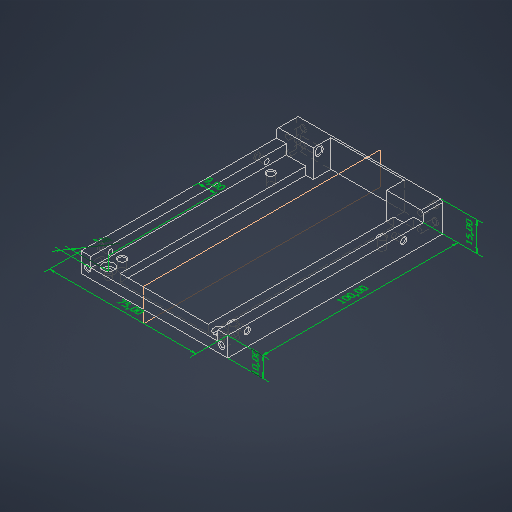
# Autodesk Inventor part: podstawa
Saved by Autodesk Inventor 2026.1 (Build 301233020, 233B)
## iProperties
Created: 2025-11-03
Part Number: podstawa
Material: Stainless Steel, Polished
Document SubType Name: Modeling
Designer: Jan
Density: 8 g/cm^3
Appearance: Stainless - Polished
Author: Jan
Autodesk Inventor part; units mm, degrees
ref_plane "YZ Plane" through (0, 0, 0) normal (1, 0, 0) x (0, 1, 0)
ref_plane "XZ Plane" through (0, 0, 0) normal (0, 1, 0) x (-1, 0, 0)
ref_plane "XY Plane" through (0, 0, 0) normal (0, 0, 1) x (1, 0, 0)
sketch "Sketch1" plane through (0, 0, 0) normal (0, 1, 0) x (-1, 0, 0)
  line L0 (37.5, 55) -> (-37.5, 55)
  line L1 (-37.5, 55) -> (-37.5, -55)
  line L2 (-37.5, -55) -> (37.5, -55)
  line L3 (37.5, -55) -> (37.5, 55)
  point P0 (0, 0)
  point P1 (0, 55)
  dimension "d1" = 75
  dimension "d2" = 37.5
  dimension "d3" = 55
  dimension "d125" = 55
  dimension "d126" = 110
  constraints: 8 end point, 2 parallel, 1 horizontal, 1 midpoint, 1 perpendicular
  measures "d1" distance of L1.end L2.end
  measures "d2" distance from line of point (0, 0) L1
  measures "d3" distance of point (0, 55) point (0, 0)
  measures "d125" distance from line of point (0, 0) L0
  measures "d126" distance of L2.end L0.start
extrude "Extrusion1" add sketch "Sketch1" along normal blind 5
sketch "Sketch2" plane through (0, 5, 0) normal (0, 1, 0) x (1, 0, 0)
  line L0 (37.5, -55) -> (37.5, 55) projected
  line L1 (37.5, -55) -> (37.5, 55)
  line L2 (37.5, 55) -> (-37.5, 55)
  line L3 (-37.5, 55) -> (-37.5, -55) projected
  line L4 (-37.5, 55) -> (-37.5, -55)
  line L5 (-37.5, -55) -> (37.5, -55) projected
  line L6 (-37.5, -55) -> (-32.5, -55)
  line L7 (-32.5, -55) -> (-32.5, 45)
  line L8 (-32.5, 45) -> (-37.5, 45)
  line L9 (-37.5, 45) -> (-37.5, -55)
  line L10 (37.5, -55) -> (32.5, -55)
  line L11 (32.5, -55) -> (32.5, 45)
  line L12 (32.5, 45) -> (37.5, 45)
  line L13 (37.5, 45) -> (37.5, -55)
  point P0 (37.5, 45)
  point P1 (-37.5, 45)
  dimension "d13" = 5
  dimension "d14" = 100
  dimension "d15" = 5
  constraints: 22 end point, 6 equal length, 3 perpendicular, 2 horizontal
  measures "d13" distance of L8.end L7.end
  measures "d14" distance of L6.end L7.end
  measures "d15" distance of L11.end L12.end
extrude "Extrusion2" add sketch "Sketch2" along normal blind 5 contours L5 L11 L12 L0 | L5 L3 L8 L7
sketch "Sketch3" plane through (0, 5, 0) normal (0, 1, 0) x (1, 0, 0)
  line L0 (-37.5, 55) -> (37.5, 55)
  line L1 (37.5, 55) -> (37.5, 45)
  line L2 (37.5, 45) -> (-37.5, 45)
  line L3 (-37.5, 45) -> (-37.5, 55)
  point P0 (0, 0)
  constraints: 8 end point, 2 parallel, 1 horizontal, 1 perpendicular
extrude "Extrusion3" add sketch "Sketch3" along normal blind 10
chamfer "Chamfer2" distance 1 angle 45 1 edges at (-37.5, 15, -50)
chamfer "Chamfer3" distance 1 angle 45 1 edges at (37.5, 15, -50)
sketch "Sketch5" plane through (-32.5, 5, -45) normal (0, 0, 1) x (1, 0, 0)
  line L0 (-4, 10) -> (69, 10) projected
  line L1 (13.75, 10) -> (51.25, 10)
  line L2 (51.25, 10) -> (51.25, 0)
  line L3 (51.25, 0) -> (13.75, 0)
  line L4 (13.75, 0) -> (13.75, 10)
  line L5 (65, 0) -> (0, 0) projected
  line L6 (-5, 5) -> (-5, 9) projected
  point P0 (32.5, -5)
  point P1 (70, 5)
  point P2 (70, 9)
  dimension "d46" = 37.5
  dimension "d47" = 10
  dimension "d48" = 10
  dimension "d49" = 18.75
  dimension "d50" = 75
  dimension "d51" = 18.75
  constraints: 8 end point, 2 parallel, 1 horizontal, 1 perpendicular, 1 point on line
  measures "d46" distance of L2.end L3.end
  measures "d47" distance of L1.start L3.end
  measures "d48" distance between parallel lines of L0 L5
  measures "d49" distance from line of L6 L1.start
  measures "d50" distance of point (70, 5) L6.start
  measures "d51" horizontal distance of point (70, 9) L1.end
extrude "Extrusion4" cut sketch "Sketch5" against normal through all
sketch "Sketch6" plane through (0, 5, 0) normal (0, 1, 0) x (1, 0, 0)
  circle A0 centre (28.5, -43) radius 2
  line L0 (-32.5, -55) -> (32.5, -55) projected
  line L1 (37.5, -55) -> (37.5, 45) projected
  line L2 (0, 0) -> (12.9632, 0) construction
  line L3 (0, 0) -> (0, -9.2072) construction
  circle A1 centre (-28.5, -43) radius 2
  circle A2 centre (28.5, 33) radius 2 construction
  circle A3 centre (-28.5, 33) radius 2 construction
  line L4 (18.75, 45) -> (36.5, 45) projected
  line L5 (-18.75, 55) -> (18.75, 55) projected
  dimension "d60" = 12
  dimension "d61" = 9
  dimension "d62" = 4
  dimension "d63" = 4
  dimension "d64" = 4
  dimension "d155" = 12
  dimension "d169" = 22
  constraints: 4 centre point, 4 end point, 2 vertical alignment, 1 horizontal, 1 horizontal alignment, 1 symmetric about line, 1 vertical, 1 other
  measures "d60" distance from line of L0 A0.centre
  measures "d61" distance from line of L1 A0.centre
  measures "d62" diameter of A0
  measures "d63" diameter of A2
  measures "d64" diameter of A3
  measures "d155" distance from line of L4 A2.centre
  measures "d169" distance from line of L5 A2.centre
hole "Hole2" at (28.5, 5, -33) at (-28.5, 5, -33) at (28.5, 5, 43) at (-28.5, 5, 43) direction (0, -1, 0) diameter 3.4587 end through all thread size "M4x0.5" class "6H" standard "ISO Metric profile"
chamfer "Chamfer4" distance 0.4 angle 45 4 edges at (-28.5, 5, -34.7294) (28.5, 5, -34.7294) (28.5, 5, 41.2706) (-28.5, 5, 41.2706)
sketch "Sketch8" plane through (37.5, 0, -55) normal (0, 0, -1) x (-1, 0, 0)
  circle A0 centre (3.75, 11.25) radius 2
  circle A1 centre (3.75, 3.75) radius 2
  line L0 (1, 15) -> (74, 15) projected
  line L1 (0, 0) -> (75, 0) projected
  line L2 (0, 0) -> (0, 14) projected
  line L3 (37.5, 0) -> (37.5, 8.4159) construction
  circle A2 centre (71.25, 11.25) radius 2
  circle A3 centre (71.25, 3.75) radius 2
  point P0 (18.75, 15)
  dimension "d90" = 4
  dimension "d91" = 4
  dimension "d92" = 3.75
  dimension "d93" = 3.75
  dimension "d94" = 3.75
  constraints: 4 centre point, 2 end point, 2 symmetric about line, 1 vertical, 1 vertical alignment, 2 other
  measures "d90" diameter of A0
  measures "d91" diameter of A1
  measures "d92" distance from line of L0 A0.centre
  measures "d93" distance from line of A1.centre L1
  measures "d94" distance from line of L2 A0.centre
hole "Hole4" at (33.75, 11.25, -55) at (33.75, 3.75, -55) at (-33.75, 11.25, -55) at (-33.75, 3.75, -55) direction (0, 0, 1) diameter 2.459 depth 8 tip angle 118 thread size "M3x0.5" class "6H" standard "ISO Metric profile"
chamfer "Chamfer6" distance 0.4 angle 45 4 edges at (33.75, 10.0205, -55) (33.75, 2.5205, -55) (-33.75, 10.0205, -55) (-33.75, 2.5205, -55)
sketch "Sketch9" plane through (0, 5, 0) normal (0, 1, 0) x (1, 0, 0)
  line L0 (22.5, -50) -> (-22.5, -50)
  line L1 (-22.5, -50) -> (-22.5, 45)
  line L2 (-22.5, 45) -> (22.5, 45)
  line L3 (22.5, 45) -> (22.5, -50)
  line L4 (37.5, -55) -> (37.5, 45) projected
  point P0 (0, 0)
  dimension "d105" = 45
  dimension "d107" = 15
  dimension "d145" = 5
  constraints: 8 end point, 2 parallel, 1 horizontal, 1 perpendicular
  measures "d105" distance of L1.end L2.end
  measures "d107" distance between parallel lines of L3 L4
  measures "d145" vertical distance of L0.start L4.start
extrude "Extrusion5" cut sketch "Sketch9" against normal blind 4
sketch "Sketch10" plane through (37.5, 0, 55) normal (1, 0, 0) x (0, 0, -1)
  circle A0 centre (10, 7) radius 2
  circle A1 centre (90, 7) radius 2
  line L0 (0, 0) -> (110, 0) projected
  line L1 (0, 0) -> (0, 10) projected
  point P0 (55, 0)
  dimension "d113" = 4
  dimension "d114" = 4
  dimension "d115" = 80
  dimension "d116" = 7
  dimension "d117" = 10
  constraints: 2 centre point, 1 horizontal alignment
  measures "d113" diameter of A0
  measures "d114" diameter of A1
  measures "d115" distance of A1.centre A0.centre
  measures "d116" distance from line of A0.centre L0
  measures "d117" distance from line of L1 A0.centre
ref_plane "Work Plane1" through (0, 5, 55) normal (1, 0, 0) x (0, 0, -1)
hole "Hole5" at (37.5, 7, 45) at (37.5, 7, -35) direction (-1, 0, 0) diameter 2.459 depth 8.8 tip angle 118 thread size "M3x0.5" class "6H" standard "ISO Metric profile"
mirror "Mirror1" about plane through (0, 5, 55) normal (1, 0, 0) of "Hole5"
sketch "Sketch11" plane through (0, 5, 0) normal (0, 1, 0) x (1, 0, 0)
  line L0 (-18.75, 45) -> (-18.75, 55) projected
  line L1 (18.75, 55) -> (18.75, 45) projected
  line L2 (-18.75, 45) -> (18.75, 45)
  line L3 (18.75, 45) -> (18.75, 55)
  line L4 (18.75, 55) -> (-18.75, 55)
  line L5 (-18.75, 55) -> (-18.75, 45)
  point P0 (0, 0)
  constraints: 8 end point, 2 parallel, 1 horizontal, 1 perpendicular
extrude "Extrusion6" cut sketch "Sketch11" against normal through all
sketch "Sketch12" plane through (-18.75, 0, -55) normal (1, 0, 0) x (0, 0, -1)
  circle A0 centre (-7, 12) radius 2
  line L0 (0, 15) -> (0, 0) projected
  line L1 (-10, 15) -> (0, 15) projected
  line L2 (-10, 1) -> (-10, 15) projected
  line L3 (0, 0) -> (-10, 0) projected
  point P0 (-55, 0)
  point P1 (-10, 5)
  dimension "d129" = 4
  dimension "d142" = 3
  dimension "d143" = 12
  dimension "d144" = 15
  constraints: 1 centre point
  measures "d129" diameter of A0
  measures "d142" distance from line of L2 A0.centre
  measures "d143" distance from line of L3 A0.centre
  measures "d144" distance of L0.end L0.start
hole "Hole6" at (-18.75, 12, -48) direction (-1, 0, 0) diameter 3.4587 depth 11 tip angle 118 thread size "M4x0.5" class "6H" standard "ISO Metric profile"
chamfer "Chamfer9" distance 0.4 angle 45 1 edges at (-18.75, 12, -46.2706)
sketch "Sketch13" plane through (-18.75, 0, -55) normal (1, 0, 0) x (0, 0, -1)
  line L0 (0, 0) -> (-10, 0) projected
  line L1 (0, 0) -> (-10, 0)
  line L2 (-10, 1) -> (-10, 0) projected
  line L3 (-10, 0) -> (-10, 1)
  line L4 (-10, 1) -> (-1, 1)
  line L5 (-1, 1) -> (-1, 15)
  line L6 (-10, 15) -> (0, 15) projected
  line L7 (0, 15) -> (0, 0)
  point P0 (-55, 0)
  dimension "d152" = 9
  constraints: 10 end point, 2 perpendicular, 1 collinear, 1 parallel, 1 point on line
  measures "d152" distance of L2.start L4.end
extrude "Extrusion7" add sketch "Sketch13" along normal blind 37.5
sketch "Sketch14" plane through (-37.5, 0, 55) normal (0, 0, 1) x (1, 0, 0)
  circle A0 centre (3.2, 4) radius 1.5
  line L0 (0, 0) -> (75, 0) projected
  line L1 (0, 0) -> (0, 10) projected
  line L2 (37.5, 0) -> (37.5, 5) construction
  circle A1 centre (71.8, 4) radius 1.5
  dimension "d156" = 3
  dimension "d157" = 4
  dimension "d158" = 3.2
  constraints: 2 centre point, 2 end point, 1 symmetric about line, 1 vertical, 1 other
  measures "d156" diameter of A0
  measures "d157" distance from line of L0 A0.centre
  measures "d158" distance from line of L1 A0.centre
hole "Hole7" at (-34.3, 4, 55) at (34.3, 4, 55) direction (0, 0, -1) diameter 2.459 depth 8 tip angle 118 thread size "M3x0.5" class "6H" standard "ISO Metric profile"
chamfer "Chamfer10" distance 0.4 angle 45 2 edges at (-34.3, 5.2295, 55) (34.3, 5.2295, 55)
sketch "Sketch15" plane through (0, 5, 0) normal (0, 1, 0) x (1, 0, 0)
  circle A0 centre (-28.5, -50) radius 2
  line L0 (0, -4.7848) -> (0, 5.6914) construction
  line L1 (-32.5, -55) -> (-32.5, 45) projected
  line L2 (-32.5, -55) -> (32.5, -55) projected
  circle A1 centre (28.5, -50) radius 2
  point P0 (0, 0)
  dimension "d170" = 4
  dimension "d171" = 4
  dimension "d172" = 5
  constraints: 2 centre point, 2 end point, 1 symmetric about line, 1 vertical, 1 other
  measures "d170" diameter of A0
  measures "d171" distance from line of L1 A0.centre
  measures "d172" distance from line of L2 A0.centre
hole "Hole8" at (-28.5, 5, 50) at (28.5, 5, 50) direction (0, -1, 0) diameter 3.2 end through all counterbore diameter 6 counterbore depth 2
chamfer "Chamfer11" distance 0.4 angle 45 4 edges at (37.5, 7, -33.7705) (37.5, 7, 46.2295) (-37.5, 7, -33.7705) (-37.5, 7, 46.2295)
equation "\"d2\" = 0.5 * d1"
equation "\"d3\" = 0.5 * d0"
equation "\"d47\" = d48"
equation "\"d49\" = 0.25 * d50"
equation "\"d94\" = d92"
equation "\"d0\" = 110"
body "Solid1"
